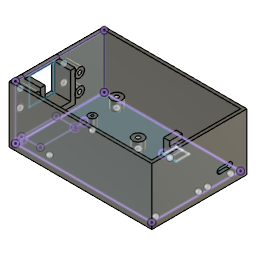
blindaphone box v1 bottom (Autodesk Fusion 360 design; units mm, degrees)
part number: 2026-05-01-20-35-57-796
Autodesk Fusion 360 part; units mm, degrees
note: some values were not read from the file. Set by a fixed rule: which face or edge a step refers to.
sketch "Sketch2" plane through (0, 0, 0) normal (0, 0, 1) x (1, 0, 0)
  line L0 (45, -30) -> (-45, -30)
  line L1 (-45, -30) -> (-45, 30)
  line L2 (-45, 30) -> (45, 30)
  line L3 (45, 30) -> (45, -30)
  line L4 (45, -30) -> (-45, 30) construction
  line L5 (-45, -30) -> (45, 30) construction
  dimension "d3" = 90
  dimension "d4" = 60
  constraint horizontal L0
  constraint perpendicular L0 L1
  constraint parallel L0 L2
  constraint parallel L1 L3
  constraint coincident L4 origin
  constraint coincident L5 origin
  measures "d3" distance of L1.end L2.end
  measures "d4" distance of L0.end L1.end
extrude "Extrude1" add sketch "Sketch2" along normal blind 36 makes body 1
shell "Shell1" thickness 2 removed faces 1 at (15, -10, 36) on bodies 1
sketch "Sketch3" plane through (-43, 0, 0) normal (1, 0, 0) x (0, 1, 0)
  line L0 (-28, 2) -> (28, 2)
  line L1 (28, 2) -> (28, 36)
  line L2 (28, 36) -> (-28, 36)
  line L3 (-28, 36) -> (-28, 2)
  circle A0 centre (-25, 20) radius 1.5
  circle A1 centre (-24.9926, 30.5) radius 1.5
  circle A2 centre (2.5074, 30.5) radius 1.5
  circle A3 centre (2.5, 20) radius 1.5
  line L4 (-19.2426, 34.5) -> (-3.2426, 34.5)
  line L5 (-3.2426, 34.5) -> (-3.2426, 17.5)
  line L6 (-3.2426, 17.5) -> (-19.2426, 17.5)
  line L7 (-19.2426, 17.5) -> (-19.2426, 34.5)
  dimension "d8" = 3
  dimension "d9" = 18
  dimension "d10" = 3
  dimension "d11" = 3
  dimension "d12" = 10.5
  dimension "d13" = 3
  dimension "d14" = 3
  dimension "d15" = 27.5
  dimension "d16" = 27.5
  dimension "d17" = 10.5
  dimension "d18" = 18
  dimension "d19" = 16
  dimension "d20" = 17
  dimension "d21" = 4
  dimension "d22" = 5.75
  dimension "d23" = 5.75
  constraint horizontal L4
  constraint vertical L5
  constraint horizontal L6
  constraint vertical L7
  measures "d8" diameter of A0
  measures "d9" distance of L0 A0.centre
  measures "d10" distance of L3 A0.centre
  measures "d11" diameter of A1
  measures "d12" distance of A0.centre A1.centre
  measures "d13" diameter of A2
  measures "d14" diameter of A3
  measures "d15" distance of A1.centre A2.centre
  measures "d16" distance of A0.centre A3.centre
  measures "d17" distance of A2.centre A3.centre
  measures "d18" distance of L0 A3.centre
  measures "d19" distance of L4.start L4.end
  measures "d20" distance of L4.start L6.end
  measures "d21" distance of A1.centre L4
  measures "d22" distance of A1.centre L7
  measures "d23" distance of A2.centre L5
extrude "Extrude2" add sketch "Sketch3" along normal blind 10 separate body contours L4 L5 L6 L7 makes body 2
shell "Shell2" thickness 3 outward yes removed faces 1 at (-33, -13.9093, 28.8333) on bodies 2
extrude "Extrude3" cut 1 faces at (-46, -7.576, 29.8333) along direction (1, 0, 0) blind 1 on bodies 2 bodies 2
extrude "Extrude4" cut sketch "Sketch3" against normal blind 3 contours L4 L5 L6 L7 bodies 1 2
sketch "Sketch13" plane through (0, 0, 37.5) normal (0, 0, 1) x (-1, 0, 0)
  line L0 (45, 0.2426) -> (45, 22.2426)
  line L1 (45, 22.2426) -> (33, 22.2426)
  line L2 (33, 22.2426) -> (33, 0.2426)
  line L3 (33, 0.2426) -> (45, 0.2426)
  line L4 (33, 0.2426) -> (43, 0.2426)
  line L5 (43, 0.2426) -> (43, 22.2426)
  line L6 (43, 22.2426) -> (33, 22.2426)
  line L7 (33, 22.2426) -> (33, 0.2426)
  dimension "d101" = 10
  constraint horizontal L4
  constraint vertical L5
  constraint horizontal L6
  constraint vertical L7
  constraint coincident L2.end L3.start
  measures "d101" distance of L2.end L4.end
extrude "Extrude14" cut sketch "Sketch13" against normal blind 3 contours L1 L2 L3 L4 L5 L6 L7 bodies 2
extrude "Extrude15" cut 1 faces at (-44.3333, -14.9093, 37.5) along direction (0, 0, -1) blind 1.5 on bodies 2 bodies 2
extrude "Extrude5" add sketch "Sketch3" along normal blind 10 separate body contours A0 | A1 | A2 | A3 makes body 3 at (-36.3333, -26.4852, 30.3506) makes body 4 at (-36.3333, -26.4925, 19.8506) makes body 5 at (-36.3333, 4.0055, 30.4252) makes body 6 at (-36.3333, 1.0075, 19.8506)
shell "Shell3" thickness 1.5 outward yes removed faces 4 at (-33, -25.2426, 31.4963) at (-33, -25.2874, 20.9316) at (-33, 2.3247, 30.9654) at (-33, 2.25, 19.1331) on bodies 3 4 5 6
sketch "Sketch4" plane through (0, 0, 2) normal (0, 0, 1) x (-1, 0, 0)
  line L0 (-43, -28) -> (43, -28)
  line L1 (43, -28) -> (43, 28)
  line L2 (43, 28) -> (-43, 28)
  line L3 (-43, 28) -> (-43, -28)
  circle A0 centre (26, 23.5) radius 0.9
  circle A1 centre (26, -3.5) radius 0.9
  circle A2 centre (-41, 23.5) radius 0.9
  circle A3 centre (-41, -3.5) radius 0.9
  line L4 (43, 26.4926) -> (43, 23.4926)
  line L5 (45, 0.2426) -> (45, 22.2426)
  line L6 (45, 22.2426) -> (33, 22.2426)
  line L7 (33, 22.2426) -> (33, 0.2426)
  line L8 (33, 0.2426) -> (45, 0.2426)
  line L9 (33, 0.4926) -> (33, -5.5074)
  dimension "d34" = 1.8
  dimension "d35" = 1.8
  dimension "d36" = 1.8
  dimension "d37" = 1.8
  dimension "d38" = 27
  dimension "d39" = 27
  dimension "d40" = 67
  dimension "d41" = 67
  dimension "d42" = 4.5
  dimension "d43" = 4.5
  dimension "d44" = 17
  dimension "d94" = 17
  measures "d34" diameter of A0
  measures "d35" diameter of A1
  measures "d36" diameter of A2
  measures "d37" diameter of A3
  measures "d38" vertical distance of A0.centre A1.centre
  measures "d39" vertical distance of A2.centre A3.centre
  measures "d40" distance of A0.centre A2.centre
  measures "d41" distance of A1.centre A3.centre
  measures "d42" distance of L2 A0.centre
  measures "d43" distance of L2 A2.centre
  measures "d44" distance of A0.centre L4
  measures "d94" distance of L1 A1.centre
extrude "Extrude6" add sketch "Sketch4" along normal blind 8 separate body contours A0 | A1 | A2 | A3 makes body 7 at (-25.3716, 4.1443, 7.3333) makes body 8 at (40.6298, -24.3204, 7.3333) makes body 9 at (-26.8989, -23.4551, 7.3333) makes body 10 at (40.6298, 4.3204, 4.6667)
shell "Shell4" thickness 1.5 outward yes removed faces 4 at (-26.1646, 3.3043, 10) at (40.9332, -23.2075, 10) at (-26.2776, -23.2008, 10) at (40.3598, 3.6859, 10) on bodies 7 8 9 10
thread "Thread1" "ISO Metric profile 1.8 M1.8x0.35 M1.8x0.35 6H" major diameter 1.8678 minor diameter 1.4711 pitch 0.35 angle 60 resizes the face on face at (40.6298, 4.3204, 4.6667) from (41, 3.5, 4) to (41, 3.5, 10) on face at (-26.8989, -23.4551, 7.3333) from (-26, -23.5, 4) to (-26, -23.5, 10) on face at (-25.3716, 4.1443, 7.3333) from (-26, 3.5, 4) to (-26, 3.5, 10) on face at (40.6298, -24.3204, 7.3333) from (41, -23.5, 4) to (41, -23.5, 10) on bodies 7 8 9 10
thread "Thread2" "ISO Metric profile 3.0 M3x0.5 M3x0.5 6H" major diameter 3.086 minor diameter 2.529 pitch 0.5 angle 60 resizes the face on face at (-36.3333, -26.4852, 30.3506) from (-39, -24.9926, 30.5) to (-33, -24.9926, 30.5) on face at (-36.3333, 4.0055, 30.4252) from (-39, 2.5074, 30.5) to (-33, 2.5074, 30.5) on face at (-36.3333, 1.0075, 19.8506) from (-39, 2.5, 20) to (-33, 2.5, 20) on face at (-36.3333, -26.4925, 19.8506) from (-39, -25, 20) to (-33, -25, 20) on bodies 3 4 5 6
sketch "Sketch6" plane through (0, 0, 2) normal (0, 0, 1) x (-1, 0, 0)
  line L0 (-43, -28) -> (43, -28)
  line L1 (43, -28) -> (43, 28)
  line L2 (43, 28) -> (-43, 28)
  line L3 (-43, 28) -> (-43, -28)
  circle A0 centre (-41.2, -23.5) radius 0.9
  circle A1 centre (-41.2, -9) radius 0.9
  line L4 (-13.4, -21) -> (-17.4, -21)
  line L5 (-17.4, -21) -> (-17.4, -13)
  line L6 (-17.4, -13) -> (-13.4, -13)
  line L7 (-13.4, -21) -> (-9.4, -21)
  line L8 (-9.4, -21) -> (-9.4, -13)
  line L9 (-9.4, -13) -> (-13.4, -13)
  line L10 (-17.4, -21) -> (-9.4, -21)
  line L11 (-9.4, -21) -> (-9.4, -13)
  line L12 (-9.4, -13) -> (-17.4, -13)
  line L13 (-17.4, -13) -> (-17.4, -21)
  line L14 (-9.4, -21) -> (-13.2, -21)
  line L15 (-13.2, -21) -> (-13.2, -13)
  line L16 (-13.2, -13) -> (-9.4, -13)
  line L17 (-9.4, -13) -> (-9.4, -21)
  dimension "d52" = 1.8
  dimension "d53" = 1.8
  dimension "d54" = 4.5
  dimension "d55" = 14.5
  dimension "d56" = 1.8
  dimension "d57" = 1.8
  dimension "d59" = 8
  dimension "d61" = 7
  dimension "d63" = 23.8
  dimension "d64" = 8
  dimension "d70" = 3.8
  constraint horizontal L4
  constraint vertical L5
  constraint horizontal L6
  constraint horizontal L7
  constraint vertical L8
  constraint horizontal L9
  constraint horizontal L10
  constraint vertical L11
  constraint horizontal L12
  constraint vertical L13
  constraint horizontal L14
  constraint vertical L15
  constraint horizontal L16
  constraint vertical L17
  measures "d52" diameter of A0
  measures "d53" diameter of A1
  measures "d54" distance of L0 A0.centre
  measures "d55" vertical distance of A0.centre A1.centre
  measures "d56" distance of L3 A0.centre
  measures "d57" distance of L3 A1.centre
  measures "d59" distance of L4.start L6.end
  measures "d61" distance of L0 L4
  measures "d63" distance of A0.centre L5
  measures "d64" distance of L8 L13
  measures "d70" distance of L7.end L14.end
extrude "Extrude7" add sketch "Sketch6" along normal blind 6 separate body contours A0 | A1 | L4 L5 L6 L7 L9 L10 L12 L13 L15 | L7 L8 L9 L10 L11 L12 L14 L15 L16 L17 makes body 11 at (13.4, 18.3333, 2) makes body 12 at (40.8298, 22.6796, 6) makes body 13 at (40.8298, 8.1796, 6)
shell "Shell5" thickness 1 outward yes removed faces 2 at (41.1332, 23.7925, 8) at (40.5598, 9.1859, 8) on bodies 12 13
thread "Thread3" "ISO Metric profile 1.8 M1.8x0.35 M1.8x0.35 6H" major diameter 1.8678 minor diameter 1.4711 pitch 0.35 angle 60 resizes the face on face at (40.8298, 22.6796, 6) from (41.2, 23.5, 3) to (41.2, 23.5, 8) on face at (40.8298, 8.1796, 6) from (41.2, 9, 3) to (41.2, 9, 8) on bodies 12 13
extrude "Extrude8" add sketch "Sketch6" along normal blind 9 contours L7 L8 L9 L10 L11 L12 L14 L15 L16 L17 bodies 11
sketch "Sketch7" plane through (0, 0, 2) normal (0, 0, 1) x (-1, 0, 0)
  line L0 (-43, -28) -> (43, -28)
  line L1 (43, -28) -> (43, 28)
  line L2 (43, 28) -> (-43, 28)
  line L3 (-43, 28) -> (-43, -28)
  circle A0 centre (1.6, -8) radius 1.5
  line L4 (-9.4, -21) -> (-9.4, -13)
  line L5 (-43, -28) -> (43, -28)
  circle A1 centre (30.6, -23.5) radius 1.5
  dimension "d73" = 3
  dimension "d74" = 11
  dimension "d75" = 20
  dimension "d76" = 3
  dimension "d77" = 4.5
  dimension "d78" = 29
  measures "d73" diameter of A0
  measures "d74" distance of A0.centre L4
  measures "d75" distance of A0.centre L5
  measures "d76" diameter of A1
  measures "d77" distance of L0 A1.centre
  measures "d78" horizontal distance of A0.centre A1.centre
sketch "Sketch9" plane through (43, 0, 0) normal (-1, 0, 0) x (0, -1, 0)
  line L0 (-28, 2) -> (28, 2)
  line L1 (28, 2) -> (28, 36)
  line L2 (28, 36) -> (-28, 36)
  line L3 (-28, 36) -> (-28, 2)
  circle A0 centre (-19, 10.7) radius 1.5
  circle A1 centre (-13, 10.7) radius 1.5
  line L4 (-13, 2) -> (-21, 2)
  line L5 (-19, 12.2) -> (-13, 12.2)
  line L6 (-13, 12.2) -> (-13, 9.2)
  line L7 (-13, 9.2) -> (-19, 9.2)
  line L8 (-19, 9.2) -> (-19, 12.2)
  circle A2 centre (-19, 10.7) radius 1.8
  circle A3 centre (-13, 10.7) radius 1.8
  line L9 (-19, 12.5) -> (-12.9659, 12.5)
  line L10 (-12.9659, 12.5) -> (-12.9659, 8.9003)
  line L11 (-12.9659, 8.9003) -> (-19, 8.9003)
  line L12 (-19, 8.9003) -> (-19, 12.5)
  dimension "d84" = 3
  dimension "d85" = 9
  dimension "d86" = 3
  dimension "d87" = 6
  dimension "d88" = 8.7
  dimension "d89" = 3.6
  dimension "d90" = 3.6
  constraint horizontal L5
  constraint vertical L6
  constraint horizontal L7
  constraint vertical L8
  constraint coincident A1 L6.end
  constraint coincident A0 L5.start
  constraint concentric A0 A2
  constraint concentric A1 A3
  constraint horizontal L9
  constraint vertical L10
  constraint horizontal L11
  constraint vertical L12
  constraint coincident A3 L10.end
  constraint coincident A2 L9.start
  measures "d84" diameter of A0
  measures "d85" distance of L3 A0.centre
  measures "d86" diameter of A1
  measures "d87" distance of A0.centre A1.centre
  measures "d88" distance of A0.centre L4
  measures "d89" diameter of A2
  measures "d90" diameter of A3
extrude "Extrude10" cut sketch "Sketch9" against normal blind 3 contours A0 L8 L12 | A0 L5 L7 A2 | A0 L8 L12 | L5 A2 L12 | A0 A2 L12 | L7 A2 L12 | L7 A2 A3 L11 | A1 A3 L10 | L5 A2 A3 L9 | L5 L7 A2 A3 | A1 L5 A3 L10 | A1 L5 L7 A3 | A1 L7 A3 L10 | A1 L6 | A1 L6 L10 | A1 L10 bodies 1
extrude "Extrude9" add sketch "Sketch7" along normal blind 6 separate body contours A0 | A1 makes body 14 at (-3.0981, 8.0748, 6) makes body 15 at (-32.0981, 23.5748, 6)
shell "Shell6" thickness 2 outward yes removed faces 2 at (-1.6012, 7.6599, 8) at (-31.0561, 23.2085, 8) on bodies 14 15
thread "Thread4" "ISO Metric profile 3.0 M3x0.5 M3x0.5 6H" major diameter 3.086 minor diameter 2.529 pitch 0.5 angle 60 resizes the face on face at (-32.0981, 23.5748, 6) from (-30.6, 23.5, 2) to (-30.6, 23.5, 8) on face at (-3.0981, 8.0748, 6) from (-1.6, 8, 2) to (-1.6, 8, 8) on bodies 14 15
